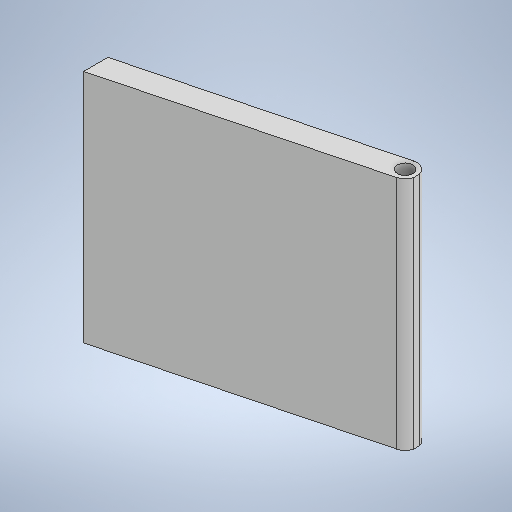
# Autodesk Inventor part: only_gate
Saved by Autodesk Inventor 2025.2 (Build 292293000, 293)
## iProperties
Created: 2025-01-19
Part Number: only_gate
Material: Типовые
Document SubType Name: Modeling
Designer: Admin
Density: 1 g/cm^3
Appearance: По умолчанию
Author: Admin
Autodesk Inventor part; units mm, degrees
ref_plane "YZ Plane" through (0, 0, 0) normal (1, 0, 0) x (0, 1, 0)
ref_plane "XZ Plane" through (0, 0, 0) normal (0, 1, 0) x (-1, 0, 0)
ref_plane "XY Plane" through (0, 0, 0) normal (0, 0, 1) x (1, 0, 0)
sketch "Эскиз1" plane through (0, 0, 0) normal (0, 1, 0) x (-1, 0, 0)
  line L0 (-53.5804, -13.9309) -> (-0.75, -0.195)
  line L1 (-52.3223, -18.77) -> (-0.75, -5.3612)
  line L2 (-55.3709, -15.7214) -> (-55.3709, -16.9796)
  circle A0 centre (-52.9514, -16.3505) radius 1.65
  line L3 (-0.75, -5.3612) -> (-0.75, -0.195)
  arc A1 (-55.3709, -16.9796) -> (-52.3223, -18.77) centre (-52.9514, -16.3505) ccw
  arc A2 (-53.5804, -13.9309) -> (-55.3709, -15.7214) centre (-52.9514, -16.3505) ccw
  point P0 (0, 0)
  constraints: 8 end point, 4 point on circle, 3 centre point, 1 coincident
extrude "Выдавливание1" add sketch "Эскиз1" along normal blind 50
